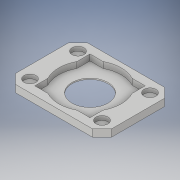
# Autodesk Inventor part: chamber_bottom
Saved by Autodesk Inventor 2019 (Build 230136000, 136)
## iProperties
Created: 2020-06-08
Part Number: chamber_bottom
Material: Generic
Document SubType Name: Modeling
Designer: honqi
Density: 1 g/cm^3
Appearance: Default
Author: honqi
Autodesk Inventor part; units mm, degrees
ref_plane "YZ Plane" through (0, 0, 0) normal (1, 0, 0) x (0, 1, 0)
ref_plane "XZ Plane" through (0, 0, 0) normal (0, 1, 0) x (-1, 0, 0)
ref_plane "XY Plane" through (0, 0, 0) normal (0, 0, 1) x (1, 0, 0)
sketch "Sketch1" plane through (0, 0, 0) normal (0, 1, 0) x (-1, 0, 0)
  line L0 (0, 0) -> (-40, 0)
  line L1 (-40, 0) -> (-40, -30)
  line L2 (-40, -30) -> (0, -30)
  line L3 (0, -30) -> (0, 0)
  dimension "d0" = 30
  dimension "d1" = 40
  constraints: 8 end point, 2 parallel, 1 horizontal, 1 perpendicular
  measures "d0" distance of L2.end L0.start
  measures "d1" distance of L1.end L2.end
extrude "Extrusion1" add sketch "Sketch1" along normal blind 3
sketch "Sketch2" plane through (0, 3, 0) normal (0, 1, 0) x (1, 0, 0)
  circle A0 centre (20, 15) radius 13
  line L0 (0, 30) -> (0, 0) projected
  line L1 (0, 0) -> (40, 0) projected
  line L2 (8.5, 3.5) -> (31.5, 3.5)
  line L3 (31.5, 3.5) -> (31.5, 26.5)
  line L4 (31.5, 26.5) -> (8.5, 26.5)
  line L5 (8.5, 26.5) -> (8.5, 3.5)
  line L6 (40, 0) -> (40, 30) projected
  dimension "d4" = 20
  dimension "d5" = 26
  dimension "d25" = 15
  dimension "d29" = 23
  dimension "d30" = 23
  dimension "d31" = 3.5
  dimension "d32" = 8.5
  constraints: 8 end point, 2 parallel, 1 centre point, 1 horizontal, 1 perpendicular
  measures "d4" distance from line of A0.centre L0
  measures "d5" diameter of A0
  measures "d25" distance from line of L1 A0.centre
  measures "d29" distance of L2.start L2.end
  measures "d30" distance of L4.end L2.start
  measures "d31" distance between parallel lines of L1 L2
  measures "d32" distance between parallel lines of L6 L3
extrude "Extrusion2" cut sketch "Sketch2" against normal blind 2.5 contours A0 L3 | L3 A0 L2 L5 L4 | L4 A0 | A0 L2 | L5 A0
sketch "Sketch3" plane through (20, 0.5, -15) normal (0, 1, 0) x (1, 0, 0)
  circle A0 centre (0, 0) radius 7.5
  point P0 (-20, -15)
  dimension "d8" = 15
  constraints: 1 centre point
  measures "d8" diameter of A0
extrude "Extrusion3" cut sketch "Sketch3" against normal blind 3.5
sketch "Sketch4" plane through (0, 3, 0) normal (0, 1, 0) x (1, 0, 0)
  circle A0 centre (5, 5) radius 2.5
  circle A1 centre (5, 25) radius 2.5
  circle A2 centre (35, 5) radius 2.5
  circle A3 centre (35, 25) radius 2.5
  circle A4 centre (20, 15) radius 7.5 projected
  point P0 (0, 0)
  dimension "d11" = 5
  dimension "d12" = 5
  dimension "d13" = 5
  dimension "d14" = 5
  dimension "d15" = 15
  dimension "d16" = 15
  dimension "d17" = 15
  dimension "d18" = 15
  dimension "d19" = 10
  dimension "d20" = 10
  dimension "d21" = 10
  dimension "d22" = 10
  constraints: 4 centre point, 1 coincident
  measures "d11" diameter of A0
  measures "d12" diameter of A1
  measures "d13" diameter of A2
  measures "d14" diameter of A3
  measures "d15" horizontal distance of A4.centre A0.centre
  measures "d16" horizontal distance of A4.centre A1.centre
  measures "d17" horizontal distance of point (20, 15) A2.centre
  measures "d18" horizontal distance of point (20, 15) A3.centre
  measures "d19" vertical distance of A0.centre point (20, 15)
  measures "d20" vertical distance of A4.centre A1.centre
  measures "d21" vertical distance of A4.centre A2.centre
  measures "d22" vertical distance of point (20, 15) A3.centre
extrude "Extrusion4" cut sketch "Sketch4" against normal blind 1.7 contours A0 | A1 | A2 | A3
chamfer "Chamfer1" distance 4 angle 45 1 edges at (40, 1.5, -30)
chamfer "Chamfer2" distance 4 angle 45 1 edges at (40, 1.5, 0)
chamfer "Chamfer3" distance 4 angle 45 1 edges at (0, 1.5, 0)
chamfer "Chamfer4" distance 4 angle 45 1 edges at (0, 1.5, -30)
sketch "Sketch5" plane through (0, 3, 0) normal (0, 1, 0) x (1, 0, 0)
  line L0 (8.5, 3.5) -> (31.5, 3.5)
  line L1 (31.5, 3.5) -> (31.5, 26.5)
  line L2 (31.5, 26.5) -> (8.5, 26.5)
  line L3 (8.5, 26.5) -> (8.5, 3.5)
  line L4 (4, 0) -> (36, 0) projected
  line L5 (40, 4) -> (40, 26) projected
  point P0 (0, 0)
  dimension "d42" = 23
  dimension "d43" = 23
  dimension "d44" = 3.5
  dimension "d45" = 8.5
  constraints: 8 end point, 2 parallel, 1 horizontal, 1 perpendicular
  measures "d42" distance of L2.end L1.end
  measures "d43" distance of L2.end L0.start
  measures "d44" distance between parallel lines of L4 L0
  measures "d45" distance between parallel lines of L5 L1
extrude "Extrusion5" cut sketch "Sketch5" against normal blind 2.5
body "Solid1"
